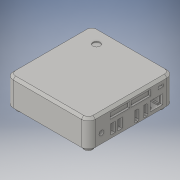
# Autodesk Inventor part: NUC
Saved by Autodesk Inventor 2016 (Build 200138000, 138)
## iProperties
Created: 2015-09-04
Part Number: NUC
Material: Generic
Document SubType Name: Modeling
Designer: lachesis
Density: 1 g/cm^3
Appearance: Default
Author: lachesis
Autodesk Inventor part; units mm, degrees
ref_plane "YZ Plane" through (0, 0, 0) normal (1, 0, 0) x (0, 1, 0)
ref_plane "XZ Plane" through (0, 0, 0) normal (0, 1, 0) x (-1, 0, 0)
ref_plane "XY Plane" through (0, 0, 0) normal (0, 0, 1) x (1, 0, 0)
sketch "Sketch1" plane through (0, 0, 0) normal (0, 1, 0) x (-1, 0, 0)
  line L0 (56.007, 58.293) -> (-56.007, 58.293)
  line L1 (-56.007, 58.293) -> (-56.007, -58.293)
  line L2 (-56.007, -58.293) -> (56.007, -58.293)
  line L3 (56.007, -58.293) -> (56.007, 58.293)
  point P0 (0, 0)
  point P1 (56.007, 0)
  point P2 (0, 58.293)
  dimension "d0" = 116.586
  dimension "d1" = 112.014
  constraints: 8 end point, 2 midpoint, 2 parallel, 1 horizontal, 1 horizontal alignment, 1 perpendicular, 1 vertical alignment
  measures "d0" distance of L2.end L0.start
  measures "d1" distance of L0.start L0.end
extrude "Extrusion1" add sketch "Sketch1" along normal blind 39.37
fillet "Fillet1" radius 9.525 4 edges at (-56.007, 19.685, 58.293) (56.007, 19.685, 58.293) (56.007, 19.685, -58.293) (-56.007, 19.685, -58.293)
chamfer "Chamfer1" distance 3.175 angle 45 8 edges at (0, 39.37, 58.293) (53.2172, 39.37, 55.5032) (56.007, 39.37, 0) (53.2172, 39.37, -55.5032) (0, 39.37, -58.293) (-53.2172, 39.37, -55.5032) (-56.007, 39.37, 0) (-53.2172, 39.37, 55.5032)
chamfer "Chamfer2" distance 3.175 angle 45 8 edges at (0, 0, 58.293) (53.2172, 0, 55.5032) (56.007, 0, 0) (53.2172, 0, -55.5032) (0, 0, -58.293) (-53.2172, 0, -55.5032) (-56.007, 0, 0) (-53.2172, 0, 55.5032)
sketch "Sketch2" plane through (56.007, 0, 48.768) normal (1, 0, 0) x (0, 0, -1)
  line L0 (20.955, 20.5486) -> (27.0764, 20.5486)
  line L1 (27.0764, 20.5486) -> (27.0764, 7.2644)
  line L2 (27.0764, 7.2644) -> (20.955, 7.2644)
  line L3 (20.955, 7.2644) -> (20.955, 20.5486)
  line L4 (-9.525, 36.195) -> (-9.525, 0) projected
  line L5 (0, 36.195) -> (97.536, 36.195) projected
  line L6 (0, 0) -> (97.536, 0) projected
  line L7 (107.061, 0) -> (107.061, 36.195) projected
  line L8 (30.6324, 20.5486) -> (36.7538, 20.5486)
  line L9 (36.7538, 20.5486) -> (36.7538, 7.2644)
  line L10 (36.7538, 7.2644) -> (30.6324, 7.2644)
  line L11 (30.6324, 7.2644) -> (30.6324, 20.5486)
  line L12 (53.9496, 19.685) -> (57.6326, 19.685)
  line L13 (57.6326, 19.685) -> (59.2836, 18.034)
  line L14 (59.2836, 18.034) -> (59.2836, 6.604)
  line L15 (59.2836, 6.604) -> (57.6326, 4.953)
  line L16 (57.6326, 4.953) -> (53.9496, 4.953)
  line L17 (53.9496, 4.953) -> (53.9496, 19.685)
  line L18 (66.1416, 19.685) -> (69.8246, 19.685)
  line L19 (69.8246, 19.685) -> (71.4756, 18.034)
  line L20 (71.4756, 18.034) -> (71.4756, 6.604)
  line L21 (71.4756, 6.604) -> (69.8246, 4.953)
  line L22 (69.8246, 4.953) -> (66.1416, 4.953)
  line L23 (66.1416, 4.953) -> (66.1416, 19.685)
  line L24 (74.7776, 20.574) -> (91.5416, 20.574)
  line L25 (91.5416, 20.574) -> (91.5416, 7.62)
  line L26 (91.5416, 7.62) -> (74.7776, 7.62)
  line L27 (74.7776, 7.62) -> (74.7776, 20.574)
  line L28 (74.7776, 9.652) -> (76.8096, 9.652)
  line L29 (76.8096, 9.652) -> (76.8096, 18.542)
  line L30 (76.8096, 18.542) -> (89.5096, 18.542)
  line L31 (89.5096, 18.542) -> (89.5096, 9.652)
  line L32 (89.5096, 9.652) -> (91.5416, 9.652)
  line L33 (89.5096, 9.652) -> (87.4776, 9.652)
  line L34 (87.4776, 9.652) -> (87.4776, 7.62)
  line L35 (76.8096, 9.652) -> (78.8416, 9.652)
  line L36 (78.8416, 9.652) -> (78.8416, 7.62)
  line L37 (85.471, 31.877) -> (92.583, 31.877)
  line L38 (92.583, 31.877) -> (92.583, 28.6258)
  line L39 (92.583, 28.6258) -> (85.471, 28.6258)
  line L40 (85.471, 28.6258) -> (85.471, 31.877)
  circle A0 centre (8.255, 16.002) radius 3.302
  line L41 (0, 3.175) -> (97.536, 3.175) projected
  point P0 (48.768, 0)
  point P1 (67.9831, 19.685)
  point P2 (55.7911, 19.685)
  dimension "d8" = 6.1214
  dimension "d9" = 13.2842
  dimension "d10" = 30.48
  dimension "d11" = 7.2644
  dimension "d12" = 13.2842
  dimension "d13" = 6.1214
  dimension "d14" = 3.556
  dimension "d15" = 135
  dimension "d16" = 135
  dimension "d18" = 5.334
  dimension "d19" = 14.732
  dimension "d20" = 17.1958
  dimension "d22" = 11.43
  dimension "d23" = 135
  dimension "d24" = 135
  dimension "d25" = 5.334
  dimension "d26" = 14.732
  dimension "d27" = 11.43
  dimension "d28" = 6.858
  dimension "d29" = 12.954
  dimension "d30" = 16.764
  dimension "d31" = 3.302
  dimension "d32" = 7.62
  dimension "d33" = 2.032
  dimension "d34" = 2.032
  dimension "d35" = 2.032
  dimension "d36" = 2.032
  dimension "d37" = 2.032
  dimension "d38" = 2.032
  dimension "d45" = 7.112
  dimension "d46" = 3.2512
  dimension "d47" = 14.478
  dimension "d48" = 4.318
  dimension "d49" = 6.604
  dimension "d50" = 12.7
  dimension "d51" = 17.78
  dimension "d96" = 1.778
  constraints: 74 end point, 16 perpendicular, 11 equal length, 7 horizontal, 7 point on line, 2 midpoint, 1 centre point, 1 horizontal alignment
  measures "d8" distance of L0.start L0.end
  measures "d9" distance of L0.end L1.end
  measures "d10" distance between parallel lines of L3 L4
  measures "d11" distance between parallel lines of L6 L2
  measures "d12" distance of L8.end L9.end
  measures "d13" distance of L8.start L8.end
  measures "d14" distance between parallel lines of L1 L11
  measures "d15" angle of L12 L13
  measures "d16" angle of L16 L15
  measures "d18" distance between parallel lines of L14 L17
  measures "d19" distance of L16.end L12.start
  measures "d20" distance between parallel lines of L17 L9
  measures "d22" distance of L13.end L14.end
  measures "d23" angle of L18 L19
  measures "d24" angle of L22 L21
  measures "d25" distance between parallel lines of L20 L23
  measures "d26" distance of L23.start L23.end
  measures "d27" distance of L19.end L20.end
  measures "d28" distance between parallel lines of L14 L23
  measures "d29" distance of L24.end L25.end
  measures "d30" distance of L24.start L24.end
  measures "d31" distance between parallel lines of L27 L20
  measures "d32" distance between parallel lines of L6 L26
  measures "d33" distance of L28.start L28.end
  measures "d34" distance between parallel lines of L24 L30
  measures "d35" distance between parallel lines of L25 L31
  measures "d36" distance between parallel lines of L26 L32
  measures "d37" distance of L31.end L33.end
  measures "d38" distance of L28.end L35.end
  measures "d45" distance of L37.start L37.end
  measures "d46" distance of L37.end L38.end
  measures "d47" distance between parallel lines of L7 L38
  measures "d48" distance between parallel lines of L5 L37
  measures "d49" diameter of A0
  measures "d50" distance edge to line of A0 L6
  measures "d51" distance from line of A0.centre L4
  measures "d96" distance between parallel lines of L41 L16
extrude "Extrusion2" cut sketch "Sketch2" against normal blind 12.7 contours L0 L1 L2 L3 | L8 L9 L10 L11 | L12 L13 L14 L15 L16 L17 | L18 L19 L20 L21 L22 L23 | L29 L30 L31 L33 L34 L26 L36 L35 | L37 L38 L39 L40 | A0
sketch "Sketch3" plane through (56.007, 0, 48.768) normal (1, 0, 0) x (0, 0, -1)
  line L0 (20.447, 33.655) -> (46.863, 33.655)
  line L1 (46.863, 33.655) -> (46.863, 26.0604)
  line L2 (46.863, 26.0604) -> (20.447, 26.0604)
  line L3 (20.447, 26.0604) -> (20.447, 33.655)
  line L4 (48.9204, 33.655) -> (75.3364, 33.655)
  line L5 (75.3364, 33.655) -> (75.3364, 26.0604)
  line L6 (75.3364, 26.0604) -> (48.9204, 26.0604)
  line L7 (48.9204, 26.0604) -> (48.9204, 33.655)
  line L8 (-9.525, 36.195) -> (-9.525, 0) projected
  line L9 (0, 36.195) -> (97.536, 36.195) projected
  line L10 (74.7776, 20.574) -> (91.5416, 20.574)
  line L11 (91.5416, 20.574) -> (91.5416, 7.62)
  line L12 (91.5416, 7.62) -> (74.7776, 7.62)
  line L13 (74.7776, 7.62) -> (74.7776, 20.574)
  line L14 (74.7776, 9.652) -> (76.8096, 9.652)
  line L15 (76.8096, 9.652) -> (76.8096, 18.542)
  line L16 (76.8096, 18.542) -> (89.5096, 18.542)
  line L17 (89.5096, 18.542) -> (89.5096, 9.652)
  line L18 (89.5096, 9.652) -> (91.5416, 9.652)
  line L19 (89.5096, 9.652) -> (87.4776, 9.652)
  line L20 (87.4776, 9.652) -> (87.4776, 7.62)
  line L21 (76.8096, 9.652) -> (78.8416, 9.652)
  line L22 (78.8416, 9.652) -> (78.8416, 7.62)
  line L23 (97.536, 36.195) -> (97.536, 0) projected
  point P0 (48.768, 0)
  dimension "d54" = 2.0574
  dimension "d55" = 7.5946
  dimension "d56" = 26.416
  dimension "d57" = 26.416
  dimension "d58" = 29.972
  dimension "d59" = 2.54
  dimension "d60" = 12.954
  dimension "d61" = 16.764
  dimension "d62" = 2.032
  dimension "d63" = 2.032
  dimension "d64" = 2.032
  dimension "d65" = 2.032
  dimension "d66" = 2.032
  dimension "d67" = 2.032
  dimension "d68" = 15.621
  dimension "d69" = 5.9944
  constraints: 42 end point, 9 perpendicular, 8 point on line, 6 parallel, 5 horizontal
  measures "d54" distance between parallel lines of L7 L1
  measures "d55" distance between parallel lines of L2 L0
  measures "d56" distance between parallel lines of L3 L1
  measures "d57" distance between parallel lines of L5 L7
  measures "d58" distance between parallel lines of L8 L3
  measures "d59" distance between parallel lines of L9 L0
  measures "d60" distance of L10.end L11.end
  measures "d61" distance of L10.start L10.end
  measures "d62" distance of L14.start L21.start
  measures "d63" distance between parallel lines of L10 L16
  measures "d64" distance between parallel lines of L11 L17
  measures "d65" distance between parallel lines of L12 L18
  measures "d66" distance of L18.start L19.end
  measures "d67" distance of L21.start L22.start
  measures "d68" distance between parallel lines of L9 L10
  measures "d69" distance between parallel lines of L23 L11
extrude "Extrusion3" cut sketch "Sketch3" against normal blind 2.54 contours L0 L1 L2 L3 | L4 L5 L6 L7 | L10 L11 L18 L17 L16 L15 L14 L13 | L14 L21 L22 L12 L13 | L11 L12 L20 L19 L18
sketch "Sketch6" plane through (0, 39.37, 0) normal (0, 1, 0) x (1, 0, 0)
  circle A0 centre (-28.702, 37.592) radius 4.826
  line L0 (-46.482, 55.118) -> (46.482, 55.118) projected
  line L1 (-52.832, -48.768) -> (-52.832, 48.768) projected
  point P0 (0, 0)
  dimension "d80" = 9.652
  dimension "d81" = 12.7
  dimension "d82" = 24.13
  constraints: 1 centre point
  measures "d80" diameter of A0
  measures "d81" distance edge to line of A0 L0
  measures "d82" distance from line of L1 A0.centre
extrude "Extrusion4" cut sketch "Sketch6" against normal blind 1.27
sketch "Sketch7" plane through (-56.007, 0, -48.768) normal (-1, 0, 0) x (0, 0, 1)
  line L0 (13.335, 18.8214) -> (26.6192, 18.8214)
  line L1 (26.6192, 18.8214) -> (26.6192, 12.7)
  line L2 (26.6192, 12.7) -> (13.335, 12.7)
  line L3 (13.335, 12.7) -> (13.335, 18.8214)
  line L4 (-9.525, 36.195) -> (-9.525, 0) projected
  line L5 (0, 0) -> (97.536, 0) projected
  point P0 (48.768, 0)
  point P1 (30.6324, 18.8214)
  dimension "d85" = 13.2842
  dimension "d86" = 6.1214
  dimension "d87" = 22.86
  dimension "d88" = 12.7
  constraints: 8 end point, 2 parallel, 1 horizontal, 1 perpendicular, 1 point on line
  measures "d85" distance of L3.end L0.end
  measures "d86" distance of L0.end L1.end
  measures "d87" distance between parallel lines of L4 L3
  measures "d88" distance between parallel lines of L5 L2
extrude "Extrusion5" cut sketch "Sketch7" against normal blind 12.7
sketch "Sketch8" plane through (0, 0, 0) normal (0, -1, 0) x (1, 0, 0)
  circle A0 centre (-45.5549, 47.8409) radius 5.6515
  line L0 (-46.482, 55.118) -> (46.482, 55.118) projected
  line L1 (-52.832, -48.768) -> (-52.832, 48.768) projected
  circle A1 centre (45.5549, -47.8409) radius 5.6515
  circle A2 centre (45.5549, 47.8409) radius 5.6515
  line L2 (52.832, 48.768) -> (52.832, -48.768) projected
  circle A3 centre (-45.5549, -47.8409) radius 5.6515
  circle A4 centre (-45.5549, 47.8409) radius 3.7719
  circle A5 centre (45.5549, 47.8409) radius 3.7719
  circle A6 centre (45.5549, -47.8409) radius 3.7719
  circle A7 centre (-45.5549, -47.8409) radius 3.7719
  point P0 (0, 0)
  dimension "d97" = 11.303
  dimension "d100" = 1.6256
  dimension "d101" = 1.6256
  dimension "d104" = 360
  dimension "d106" = 11.303
  dimension "d107" = 1.6256
  dimension "d108" = 1.6256
  dimension "d111" = 360
  dimension "d113" = 1.8796
  dimension "d114" = 1.8796
  dimension "d115" = 1.8796
  dimension "d116" = 1.8796
  constraints: 8 centre point, 4 coincident, 10 other
  measures "d97" diameter of A0
  measures "d100" distance edge to line of A0 L0
  measures "d101" distance edge to line of A0 L1
  measures "d106" diameter of A2
  measures "d107" distance edge to line of A2 L0
  measures "d108" distance edge to line of A2 L2
  measures "d113" radial gap between concentric circles of A0 A4
  measures "d114" radial gap between concentric circles of A2 A5
  measures "d115" radial gap between concentric circles of A3 A7
  measures "d116" radial gap between concentric circles of A1 A6
extrude "Extrusion6" add sketch "Sketch8" along normal blind 2.54
equation "\"d12\" = d9"
equation "\"d13\" = d8"
equation "\"d16\" = d15"
equation "\"d24\" = d23"
equation "\"d34\" = d33"
equation "\"d35\" = d33"
equation "\"d36\" = d33"
equation "\"d57\" = d56"
equation "\"d63\" = d62"
equation "\"d64\" = d62"
equation "\"d65\" = d62"
equation "\"d107\" = d100"
equation "\"d108\" = d100"
equation "\"d114\" = d113"
equation "\"d115\" = d113"
equation "\"d116\" = d113"
body "Solid1"
